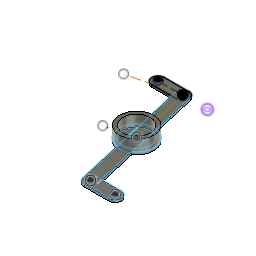
100x100 Naca 0012 airfoil w 3.8mm holes (Autodesk Fusion 360 design; units mm, degrees)
Autodesk Fusion 360 part; units mm, degrees
sketch "NACA_0012_AIRFOILS_1.0" plane through (0, 0, 0) normal (0, 0, 1) x (1, 0, 0)
  spline S0 degree 5 poles (100, 0.126) (99.9938, 0.1269) (99.9778, 0.1291) (99.9427, 0.134) (99.8738, 0.1437) (99.7628, 0.1592) (99.6406, 0.1763) (99.5101, 0.1946) (99.3691, 0.2142) (99.2177, 0.2353) (99.0577, 0.2575) (98.8912, 0.2806) (98.7187, 0.3044) (98.5403, 0.3289) (98.356, 0.3543) (98.166, 0.3804) (97.9707, 0.4072) (97.7707, 0.4346) (97.5662, 0.4625) (97.3575, 0.4909) (97.1446, 0.5198) (96.9277, 0.5491) (96.7068, 0.5789) (96.4822, 0.6091) (96.254, 0.6397) (96.0224, 0.6708) (95.7875, 0.7021) (95.5493, 0.7338) (95.3081, 0.7658) (95.0637, 0.7982) (94.8164, 0.8308) (94.5663, 0.8637) (94.3133, 0.8969) (94.0576, 0.9304) (93.7993, 0.9641) (93.5384, 0.998) (93.275, 1.0321) (93.0091, 1.0665) (92.7408, 1.101) (92.4702, 1.1357) (92.1973, 1.1706) (91.9221, 1.2057) (91.6448, 1.2409) (91.3653, 1.2763) (91.0838, 1.3119) (90.8001, 1.3476) (90.5145, 1.3835) (90.2269, 1.4194) (89.9374, 1.4555) (89.646, 1.4917) (89.3527, 1.528) (89.0576, 1.5644) (88.7607, 1.6009) (88.4621, 1.6375) (88.1617, 1.6742) (87.8597, 1.7109) (87.556, 1.7477) (87.2507, 1.7846) (86.9439, 1.8216) (86.6354, 1.8586) (86.3255, 1.8956) (86.014, 1.9327) (85.701, 1.9699) (85.3866, 2.0071) (85.0707, 2.0443) (84.7534, 2.0816) (84.4348, 2.1188) (84.1147, 2.1561) (83.7934, 2.1934) (83.4707, 2.2307) (83.1468, 2.268) (82.8216, 2.3053) (82.4952, 2.3426) (82.1675, 2.3799) (81.8386, 2.4172) (81.5086, 2.4545) (81.1774, 2.4918) (80.845, 2.5291) (80.5115, 2.5664) (80.1769, 2.6036) (79.8413, 2.6408) (79.5046, 2.6779) (79.1668, 2.715) (78.828, 2.7521) (78.4882, 2.7891) (78.1474, 2.8261) (77.8056, 2.863) (77.4628, 2.8999) (77.1192, 2.9368) (76.7745, 2.9735) (76.429, 3.0103) (76.0826, 3.0469) (75.7353, 3.0835) (75.3872, 3.1199) (75.0382, 3.1564) (74.6884, 3.1927) (74.3377, 3.229) (73.9863, 3.2652) (73.634, 3.3013) (73.281, 3.3373) (72.9273, 3.3732) (72.5728, 3.4091) (72.2175, 3.4448) (71.8616, 3.4805) (71.5049, 3.516) (71.1476, 3.5514) (70.7896, 3.5867) (70.4309, 3.6219) (70.0716, 3.657) (69.7117, 3.6919) (69.3511, 3.7268) (68.99, 3.7615) (68.6282, 3.7961) (68.2659, 3.8306) (67.903, 3.8649) (67.5395, 3.8991) (67.1755, 3.9331) (66.811, 3.967) (66.4459, 4.0007) (66.0804, 4.0343) (65.7143, 4.0678) (65.3478, 4.1011) (64.9808, 4.1342) (64.6134, 4.1672) (64.2455, 4.2001) (63.8771, 4.2327) (63.5084, 4.2652) (63.1392, 4.2975) (62.7697, 4.3296) (62.3997, 4.3616) (62.0294, 4.3933) (61.6587, 4.4249) (61.2877, 4.4563) (60.9163, 4.4874) (60.5447, 4.5184) (60.1726, 4.5492) (59.8003, 4.5798) (59.4277, 4.6101) (59.0549, 4.6403) (58.6817, 4.6702) (58.3083, 4.7) (57.9346, 4.7295) (57.5607, 4.7588) (57.1865, 4.7878) (56.8122, 4.8166) (56.4376, 4.8452) (56.0628, 4.8736) (55.6879, 4.9016) (55.3128, 4.9295) (54.9375, 4.9571) (54.5621, 4.9844) (54.1865, 5.0115) (53.8108, 5.0383) (53.435, 5.0648) (53.0591, 5.0911) (52.6831, 5.1171) (52.307, 5.1428) (51.9308, 5.1682) (51.5545, 5.1934) (51.1782, 5.2182) (50.8019, 5.2428) (50.4255, 5.2671) (50.0491, 5.291) (49.6727, 5.3147) (49.2963, 5.338) (48.9199, 5.361) (48.5435, 5.3837) (48.1672, 5.4061) (47.7909, 5.4281) (47.4146, 5.4498) (47.0384, 5.4711) (46.6623, 5.4922) (46.2863, 5.5128) (45.9104, 5.5331) (45.5345, 5.5531) (45.1588, 5.5727) (44.7833, 5.5919) (44.4078, 5.6107) (44.0326, 5.6292) (43.6574, 5.6473) (43.2825, 5.665) (42.9077, 5.6823) (42.5332, 5.6992) (42.1588, 5.7157) (41.7847, 5.7319) (41.4108, 5.7475) (41.0371, 5.7628) (40.6637, 5.7777) (40.2905, 5.7921) (39.9177, 5.8061) (39.5451, 5.8197) (39.1728, 5.8328) (38.8008, 5.8455) (38.4291, 5.8578) (38.0578, 5.8695) (37.6868, 5.8809) (37.3162, 5.8917) (36.9459, 5.9021) (36.576, 5.912) (36.2065, 5.9214) (35.8375, 5.9303) (35.4688, 5.9388) (35.1006, 5.9467) (34.7328, 5.9541) (34.3654, 5.961) (33.9986, 5.9674) (33.6322, 5.9733) (33.2662, 5.9786) (32.9008, 5.9834) (32.536, 5.9877) (32.1716, 5.9914) (31.8078, 5.9945) (31.4445, 5.9971) (31.0818, 5.9992) (30.7197, 6.0007) (30.3582, 6.0015) (29.9973, 6.0019) (29.637, 6.0016) (29.2774, 6.0007) (28.9184, 5.9992) (28.5601, 5.9972) (28.2024, 5.9945) (27.8455, 5.9912) (27.4892, 5.9873) (27.1337, 5.9828) (26.779, 5.9776) (26.4249, 5.9718) (26.0717, 5.9653) (25.7192, 5.9582) (25.3676, 5.9504) (25.0167, 5.9419) (24.6667, 5.9327) (24.3176, 5.9229) (23.9693, 5.9123) (23.6219, 5.9011) (23.2754, 5.8892) (22.9298, 5.8766) (22.5851, 5.8632) (22.2414, 5.8492) (21.8987, 5.8344) (21.5569, 5.8188) (21.2162, 5.8026) (20.8764, 5.7855) (20.5378, 5.7677) (20.2001, 5.7492) (19.8636, 5.7298) (19.5282, 5.7097) (19.1939, 5.6888) (18.8607, 5.6671) (18.5287, 5.6446) (18.1979, 5.6213) (17.8683, 5.5971) (17.5399, 5.5721) (17.2127, 5.5463) (16.8869, 5.5197) (16.5623, 5.4922) (16.2391, 5.4638) (15.9172, 5.4345) (15.5967, 5.4043) (15.2776, 5.3733) (14.9599, 5.3414) (14.6437, 5.3085) (14.3289, 5.2747) (14.0157, 5.24) (13.704, 5.2043) (13.3938, 5.1677) (13.0852, 5.1302) (12.7783, 5.0916) (12.473, 5.0521) (12.1694, 5.0116) (11.8675, 4.9701) (11.5673, 4.9276) (11.269, 4.884) (10.9725, 4.8394) (10.6779, 4.7937) (10.3851, 4.7469) (10.0943, 4.699) (9.8055, 4.65) (9.5187, 4.5999) (9.234, 4.5486) (8.9514, 4.4962) (8.6709, 4.4426) (8.3927, 4.3878) (8.1167, 4.3318) (7.843, 4.2746) (7.5717, 4.2161) (7.3029, 4.1564) (7.0365, 4.0953) (6.7727, 4.0329) (6.5114, 3.9691) (6.2529, 3.9039) (5.9971, 3.8373) (5.7442, 3.7693) (5.4941, 3.6998) (5.247, 3.6288) (5.0031, 3.5562) (4.7622, 3.4821) (4.5247, 3.4063) (4.2905, 3.3288) (4.0599, 3.2495) (3.8328, 3.1685) (3.6094, 3.0857) (3.39, 3.0009) (3.1745, 2.9142) (2.9632, 2.8254) (2.7563, 2.7345) (2.5539, 2.6415) (2.3562, 2.5461) (2.1635, 2.4483) (1.976, 2.3481) (1.794, 2.2452) (1.6177, 2.1397) (1.4475, 2.0313) (1.2838, 1.9199) (1.1269, 1.8055) (0.9774, 1.6878) (0.8357, 1.5667) (0.7024, 1.442) (0.5781, 1.3137) (0.4636, 1.1815) (0.3595, 1.0456) (0.2668, 0.9058) (0.1864, 0.7624) (0.1191, 0.6153) (0.0658, 0.4649) (0.0272, 0.3117) (0.0039, 0.1564) (-0.0039, 0) (0.0039, -0.1564) (0.0272, -0.3117) (0.0658, -0.4649) (0.1191, -0.6153) (0.1864, -0.7624) (0.2668, -0.9058) (0.3595, -1.0456) (0.4636, -1.1815) (0.5781, -1.3137) (0.7024, -1.442) (0.8357, -1.5667) (0.9774, -1.6878) (1.1269, -1.8055) (1.2838, -1.9199) (1.4475, -2.0313) (1.6177, -2.1397) (1.794, -2.2452) (1.976, -2.3481) (2.1635, -2.4483) (2.3562, -2.5461) (2.5539, -2.6415) (2.7563, -2.7345) (2.9632, -2.8254) (3.1745, -2.9142) (3.39, -3.0009) (3.6094, -3.0857) (3.8328, -3.1685) (4.0599, -3.2495) (4.2905, -3.3288) (4.5247, -3.4063) (4.7622, -3.4821) (5.0031, -3.5562) (5.247, -3.6288) (5.4941, -3.6998) (5.7442, -3.7693) (5.9971, -3.8373) (6.2529, -3.9039) (6.5114, -3.9691) (6.7727, -4.0329) (7.0365, -4.0953) (7.3029, -4.1564) (7.5717, -4.2161) (7.843, -4.2746) (8.1167, -4.3318) (8.3927, -4.3878) (8.6709, -4.4426) (8.9514, -4.4962) (9.234, -4.5486) (9.5187, -4.5999) (9.8055, -4.65) (10.0943, -4.699) (10.3851, -4.7469) (10.6779, -4.7937) (10.9725, -4.8394) (11.269, -4.884) (11.5673, -4.9276) (11.8675, -4.9701) (12.1694, -5.0116) (12.473, -5.0521) (12.7783, -5.0916) (13.0852, -5.1302) (13.3938, -5.1677) (13.704, -5.2043) (14.0157, -5.24) (14.3289, -5.2747) (14.6437, -5.3085) (14.9599, -5.3414) (15.2776, -5.3733) (15.5967, -5.4043) (15.9172, -5.4345) (16.2391, -5.4638) (16.5623, -5.4922) (16.8869, -5.5197) (17.2127, -5.5463) (17.5399, -5.5721) (17.8683, -5.5971) (18.1979, -5.6213) (18.5287, -5.6446) (18.8607, -5.6671) (19.1939, -5.6888) (19.5282, -5.7097) (19.8636, -5.7298) (20.2001, -5.7492) (20.5378, -5.7677) (20.8764, -5.7855) (21.2162, -5.8026) (21.5569, -5.8188) (21.8987, -5.8344) (22.2414, -5.8492) (22.5851, -5.8632) (22.9298, -5.8766) (23.2754, -5.8892) (23.6219, -5.9011) (23.9693, -5.9123) (24.3176, -5.9229) (24.6667, -5.9327) (25.0167, -5.9419) (25.3676, -5.9504) (25.7192, -5.9582) (26.0717, -5.9653) (26.4249, -5.9718) (26.779, -5.9776) (27.1337, -5.9828) (27.4892, -5.9873) (27.8455, -5.9912) (28.2024, -5.9945) (28.5601, -5.9972) (28.9184, -5.9992) (29.2774, -6.0007) (29.637, -6.0016) (29.9973, -6.0019) (30.3582, -6.0015) (30.7197, -6.0007) (31.0818, -5.9992) (31.4445, -5.9971) (31.8078, -5.9945) (32.1716, -5.9914) (32.536, -5.9877) (32.9008, -5.9834) (33.2662, -5.9786) (33.6322, -5.9733) (33.9986, -5.9674) (34.3654, -5.961) (34.7328, -5.9541) (35.1006, -5.9467) (35.4688, -5.9388) (35.8375, -5.9303) (36.2065, -5.9214) (36.576, -5.912) (36.9459, -5.9021) (37.3162, -5.8917) (37.6868, -5.8809) (38.0578, -5.8695) (38.4291, -5.8578) (38.8008, -5.8455) (39.1728, -5.8328) (39.5451, -5.8197) (39.9177, -5.8061) (40.2905, -5.7921) (40.6637, -5.7777) (41.0371, -5.7628) (41.4108, -5.7475) (41.7847, -5.7319) (42.1588, -5.7157) (42.5332, -5.6992) (42.9077, -5.6823) (43.2825, -5.665) (43.6574, -5.6473) (44.0326, -5.6292) (44.4078, -5.6107) (44.7833, -5.5919) (45.1588, -5.5727) (45.5345, -5.5531) (45.9104, -5.5331) (46.2863, -5.5128) (46.6623, -5.4922) (47.0384, -5.4711) (47.4146, -5.4498) (47.7909, -5.4281) (48.1672, -5.4061) (48.5435, -5.3837) (48.9199, -5.361) (49.2963, -5.338) (49.6727, -5.3147) (50.0491, -5.291) (50.4255, -5.2671) (50.8019, -5.2428) (51.1782, -5.2182) (51.5545, -5.1934) (51.9308, -5.1682) (52.307, -5.1428) (52.6831, -5.1171) (53.0591, -5.0911) (53.435, -5.0648) (53.8108, -5.0383) (54.1865, -5.0115) (54.5621, -4.9844) (54.9375, -4.9571) (55.3128, -4.9295) (55.6879, -4.9016) (56.0628, -4.8736) (56.4376, -4.8452) (56.8122, -4.8166) (57.1865, -4.7878) (57.5607, -4.7588) (57.9346, -4.7295) (58.3083, -4.7) (58.6817, -4.6702) (59.0549, -4.6403) (59.4277, -4.6101) (59.8003, -4.5798) (60.1726, -4.5492) (60.5447, -4.5184) (60.9163, -4.4874) (61.2877, -4.4563) (61.6587, -4.4249) (62.0294, -4.3933) (62.3997, -4.3616) (62.7697, -4.3296) (63.1392, -4.2975) (63.5084, -4.2652) (63.8771, -4.2327) (64.2455, -4.2001) (64.6134, -4.1672) (64.9808, -4.1342) (65.3478, -4.1011) (65.7143, -4.0678) (66.0804, -4.0343) (66.4459, -4.0007) (66.811, -3.967) (67.1755, -3.9331) (67.5395, -3.8991) (67.903, -3.8649) (68.2659, -3.8306) (68.6282, -3.7961) (68.99, -3.7615) (69.3511, -3.7268) (69.7117, -3.6919) (70.0716, -3.657) (70.4309, -3.6219) (70.7896, -3.5867) (71.1476, -3.5514) (71.5049, -3.516) (71.8616, -3.4805) (72.2175, -3.4448) (72.5728, -3.4091) (72.9273, -3.3732) (73.281, -3.3373) (73.634, -3.3013) (73.9863, -3.2652) (74.3377, -3.229) (74.6884, -3.1927) (75.0382, -3.1564) (75.3872, -3.1199) (75.7353, -3.0835) (76.0826, -3.0469) (76.429, -3.0103) (76.7745, -2.9735) (77.1192, -2.9368) (77.4628, -2.8999) (77.8056, -2.863) (78.1474, -2.8261) (78.4882, -2.7891) (78.828, -2.7521) (79.1668, -2.715) (79.5046, -2.6779) (79.8413, -2.6408) (80.1769, -2.6036) (80.5115, -2.5664) (80.845, -2.5291) (81.1774, -2.4918) (81.5086, -2.4545) (81.8386, -2.4172) (82.1675, -2.3799) (82.4952, -2.3426) (82.8216, -2.3053) (83.1468, -2.268) (83.4707, -2.2307) (83.7934, -2.1934) (84.1147, -2.1561) (84.4348, -2.1188) (84.7534, -2.0816) (85.0707, -2.0443) (85.3866, -2.0071) (85.701, -1.9699) (86.014, -1.9327) (86.3255, -1.8956) (86.6354, -1.8586) (86.9439, -1.8216) (87.2507, -1.7846) (87.556, -1.7477) (87.8597, -1.7109) (88.1617, -1.6742) (88.4621, -1.6375) (88.7607, -1.6009) (89.0576, -1.5644) (89.3527, -1.528) (89.646, -1.4917) (89.9374, -1.4555) (90.2269, -1.4194) (90.5145, -1.3835) (90.8001, -1.3476) (91.0838, -1.3119) (91.3653, -1.2763) (91.6448, -1.2409) (91.9221, -1.2057) (92.1973, -1.1706) (92.4702, -1.1357) (92.7408, -1.101) (93.0091, -1.0665) (93.275, -1.0321) (93.5384, -0.998) (93.7993, -0.9641) (94.0576, -0.9304) (94.3133, -0.8969) (94.5663, -0.8637) (94.8164, -0.8308) (95.0637, -0.7982) (95.3081, -0.7658) (95.5493, -0.7338) (95.7875, -0.7021) (96.0224, -0.6708) (96.254, -0.6397) (96.4822, -0.6091) (96.7068, -0.5789) (96.9277, -0.5491) (97.1446, -0.5198) (97.3575, -0.4909) (97.5662, -0.4625) (97.7707, -0.4346) (97.9707, -0.4072) (98.166, -0.3804) (98.356, -0.3543) (98.5403, -0.3289) (98.7187, -0.3044) (98.8912, -0.2806) (99.0577, -0.2575) (99.2177, -0.2353) (99.3691, -0.2142) (99.5101, -0.1946) (99.6406, -0.1763) (99.7628, -0.1592) (99.8738, -0.1437) (99.9427, -0.134) (99.9778, -0.1291) (99.9938, -0.1269) (100, -0.126) knots 0 0 0 0 0 0 0.00153846 0.00307692 0.00461538 0.00615385 0.00769231 0.00923077 0.01076923 0.01230769 0.01384615 0.01538462 0.01692308 0.01846154 0.02 0.02153846 0.02307692 0.02461538 0.02615385 0.02769231 0.02923077 0.03076923 0.03230769 0.03384615 0.03538462 0.03692308 0.03846154 0.04 0.04153846 0.04307692 0.04461538 0.04615385 0.04769231 0.04923077 0.05076923 0.05230769 0.05384615 0.05538462 0.05692308 0.05846154 0.06 0.06153846 0.06307692 0.06461538 0.06615385 0.06769231 0.06923077 0.07076923 0.07230769 0.07384615 0.07538462 0.07692308 0.07846154 0.08 0.08153846 0.08307692 0.08461538 0.08615385 0.08769231 0.08923077 0.09076923 0.09230769 0.09384615 0.09538462 0.09692308 0.09846154 0.1 0.10153846 0.10307692 0.10461538 0.10615385 0.10769231 0.10923077 0.11076923 0.11230769 0.11384615 0.11538462 0.11692308 0.11846154 0.12 0.12153846 0.12307692 0.12461538 0.12615385 0.12769231 0.12923077 0.13076923 0.13230769 0.13384615 0.13538462 0.13692308 0.13846154 0.14 0.14153846 0.14307692 0.14461538 0.14615385 0.14769231 0.14923077 0.15076923 0.15230769 0.15384615 0.15538462 0.15692308 0.15846154 0.16 0.16153846 0.16307692 0.16461538 0.16615385 0.16769231 0.16923077 0.17076923 0.17230769 0.17384615 0.17538462 0.17692308 0.17846154 0.18 0.18153846 0.18307692 0.18461538 0.18615385 0.18769231 0.18923077 0.19076923 0.19230769 0.19384615 0.19538462 0.19692308 0.19846154 0.2 0.20153846 0.20307692 0.20461538 0.20615385 0.20769231 0.20923077 0.21076923 0.21230769 0.21384615 0.21538462 0.21692308 0.21846154 0.22 0.22153846 0.22307692 0.22461538 0.22615385 0.22769231 0.22923077 0.23076923 0.23230769 0.23384615 0.23538462 0.23692308 0.23846154 0.24 0.24153846 0.24307692 0.24461538 0.24615385 0.24769231 0.24923077 0.25076923 0.25230769 0.25384615 0.25538462 0.25692308 0.25846154 0.26 0.26153846 0.26307692 0.26461538 0.26615385 0.26769231 0.26923077 0.27076923 0.27230769 0.27384615 0.27538462 0.27692308 0.27846154 0.28 0.28153846 0.28307692 0.28461538 0.28615385 0.28769231 0.28923077 0.29076923 0.29230769 0.29384615 0.29538462 0.29692308 0.29846154 0.3 0.30153846 0.30307692 0.30461538 0.30615385 0.30769231 0.30923077 0.31076923 0.31230769 0.31384615 0.31538462 0.31692308 0.31846154 0.32 0.32153846 0.32307692 0.32461538 0.32615385 0.32769231 0.32923077 0.33076923 0.33230769 0.33384615 0.33538462 0.33692308 0.33846154 0.34 0.34153846 0.34307692 0.34461538 0.34615385 0.34769231 0.34923077 0.35076923 0.35230769 0.35384615 0.35538462 0.35692308 0.35846154 0.36 0.36153846 0.36307692 0.36461538 0.36615385 0.36769231 0.36923077 0.37076923 0.37230769 0.37384615 0.37538462 0.37692308 0.37846154 0.38 0.38153846 0.38307692 0.38461538 0.38615385 0.38769231 0.38923077 0.39076923 0.39230769 0.39384615 0.39538462 0.39692308 0.39846154 0.4 0.40153846 0.40307692 0.40461538 0.40615385 0.40769231 0.40923077 0.41076923 0.41230769 0.41384615 0.41538462 0.41692308 0.41846154 0.42 0.42153846 0.42307692 0.42461538 0.42615385 0.42769231 0.42923077 0.43076923 0.43230769 0.43384615 0.43538462 0.43692308 0.43846154 0.44 0.44153846 0.44307692 0.44461538 0.44615385 0.44769231 0.44923077 0.45076923 0.45230769 0.45384615 0.45538462 0.45692308 0.45846154 0.46 0.46153846 0.46307692 0.46461538 0.46615385 0.46769231 0.46923077 0.47076923 0.47230769 0.47384615 0.47538462 0.47692308 0.47846154 0.48 0.48153846 0.48307692 0.48461538 0.48615385 0.48769231 0.48923077 0.49076923 0.49230769 0.49384615 0.49538462 0.49692308 0.49846154 0.5 0.50153846 0.50307692 0.50461538 0.50615385 0.50769231 0.50923077 0.51076923 0.51230769 0.51384615 0.51538462 0.51692308 0.51846154 0.52 0.52153846 0.52307692 0.52461538 0.52615385 0.52769231 0.52923077 0.53076923 0.53230769 0.53384615 0.53538462 0.53692308 0.53846154 0.54 0.54153846 0.54307692 0.54461538 0.54615385 0.54769231 0.54923077 0.55076923 0.55230769 0.55384615 0.55538462 0.55692308 0.55846154 0.56 0.56153846 0.56307692 0.56461538 0.56615385 0.56769231 0.56923077 0.57076923 0.57230769 0.57384615 0.57538462 0.57692308 0.57846154 0.58 0.58153846 0.58307692 0.58461538 0.58615385 0.58769231 0.58923077 0.59076923 0.59230769 0.59384615 0.59538462 0.59692308 0.59846154 0.6 0.60153846 0.60307692 0.60461538 0.60615385 0.60769231 0.60923077 0.61076923 0.61230769 0.61384615 0.61538462 0.61692308 0.61846154 0.62 0.62153846 0.62307692 0.62461538 0.62615385 0.62769231 0.62923077 0.63076923 0.63230769 0.63384615 0.63538462 0.63692308 0.63846154 0.64 0.64153846 0.64307692 0.64461538 0.64615385 0.64769231 0.64923077 0.65076923 0.65230769 0.65384615 0.65538462 0.65692308 0.65846154 0.66 0.66153846 0.66307692 0.66461538 0.66615385 0.66769231 0.66923077 0.67076923 0.67230769 0.67384615 0.67538462 0.67692308 0.67846154 0.68 0.68153846 0.68307692 0.68461538 0.68615385 0.68769231 0.68923077 0.69076923 0.69230769 0.69384615 0.69538462 0.69692308 0.69846154 0.7 0.70153846 0.70307692 0.70461538 0.70615385 0.70769231 0.70923077 0.71076923 0.71230769 0.71384615 0.71538462 0.71692308 0.71846154 0.72 0.72153846 0.72307692 0.72461538 0.72615385 0.72769231 0.72923077 0.73076923 0.73230769 0.73384615 0.73538462 0.73692308 0.73846154 0.74 0.74153846 0.74307692 0.74461538 0.74615385 0.74769231 0.74923077 0.75076923 0.75230769 0.75384615 0.75538462 0.75692308 0.75846154 0.76 0.76153846 0.76307692 0.76461538 0.76615385 0.76769231 0.76923077 0.77076923 0.77230769 0.77384615 0.77538462 0.77692308 0.77846154 0.78 0.78153846 0.78307692 0.78461538 0.78615385 0.78769231 0.78923077 0.79076923 0.79230769 0.79384615 0.79538462 0.79692308 0.79846154 0.8 0.80153846 0.80307692 0.80461538 0.80615385 0.80769231 0.80923077 0.81076923 0.81230769 0.81384615 0.81538462 0.81692308 0.81846154 0.82 0.82153846 0.82307692 0.82461538 0.82615385 0.82769231 0.82923077 0.83076923 0.83230769 0.83384615 0.83538462 0.83692308 0.83846154 0.84 0.84153846 0.84307692 0.84461538 0.84615385 0.84769231 0.84923077 0.85076923 0.85230769 0.85384615 0.85538462 0.85692308 0.85846154 0.86 0.86153846 0.86307692 0.86461538 0.86615385 0.86769231 0.86923077 0.87076923 0.87230769 0.87384615 0.87538462 0.87692308 0.87846154 0.88 0.88153846 0.88307692 0.88461538 0.88615385 0.88769231 0.88923077 0.89076923 0.89230769 0.89384615 0.89538462 0.89692308 0.89846154 0.9 0.90153846 0.90307692 0.90461538 0.90615385 0.90769231 0.90923077 0.91076923 0.91230769 0.91384615 0.91538462 0.91692308 0.91846154 0.92 0.92153846 0.92307692 0.92461538 0.92615385 0.92769231 0.92923077 0.93076923 0.93230769 0.93384615 0.93538462 0.93692308 0.93846154 0.94 0.94153846 0.94307692 0.94461538 0.94615385 0.94769231 0.94923077 0.95076923 0.95230769 0.95384615 0.95538462 0.95692308 0.95846154 0.96 0.96153846 0.96307692 0.96461538 0.96615385 0.96769231 0.96923077 0.97076923 0.97230769 0.97384615 0.97538462 0.97692308 0.97846154 0.98 0.98153846 0.98307692 0.98461538 0.98615385 0.98769231 0.98923077 0.99076923 0.99230769 0.99384615 0.99538462 0.99692308 0.99846154 1 1 1 1 1 1
  line L0 (100, -0.126) -> (100, 0.126)
  line L1 (0, 0) -> (100, 0) construction
  circle A0 centre (30, 0) radius 1.9
  point P0 (99.9416, 0.1342)
  point P1 (99.7666, 0.1587)
  point P2 (99.4753, 0.1994)
  point P3 (99.0685, 0.256)
  point P4 (98.5471, 0.328)
  point P5 (97.9123, 0.4152)
  point P6 (97.1656, 0.5169)
  point P7 (96.3087, 0.6324)
  point P8 (95.3437, 0.7611)
  point P9 (94.2728, 0.9022)
  point P10 (93.0985, 1.0549)
  point P11 (91.8235, 1.2182)
  point P12 (90.4509, 1.3914)
  point P13 (88.9837, 1.5735)
  point P14 (87.4255, 1.7635)
  point P15 (85.78, 1.9605)
  point P16 (84.0508, 2.1635)
  point P17 (82.2421, 2.3714)
  point P18 (80.3581, 2.5834)
  point P19 (78.4032, 2.7983)
  point P20 (76.382, 3.0152)
  point P21 (74.2992, 3.2329)
  point P22 (72.1596, 3.4506)
  point P23 (69.9682, 3.667)
  point P24 (67.7303, 3.8811)
  point P25 (65.4509, 4.0917)
  point P26 (63.1354, 4.2978)
  point P27 (60.7892, 4.498)
  point P28 (58.4179, 4.6912)
  point P29 (56.0268, 4.8762)
  point P30 (53.6217, 5.0516)
  point P31 (51.2082, 5.2162)
  point P32 (48.7918, 5.3687)
  point P33 (46.3783, 5.5077)
  point P34 (43.9732, 5.632)
  point P35 (41.5822, 5.7403)
  point P36 (39.2108, 5.8314)
  point P37 (36.8646, 5.9042)
  point P38 (34.5492, 5.9575)
  point P39 (32.2698, 5.9903)
  point P40 (30.0318, 6.0017)
  point P41 (27.8404, 5.991)
  point P42 (25.7008, 5.9576)
  point P43 (23.618, 5.9008)
  point P44 (21.5968, 5.8205)
  point P45 (19.6419, 5.7164)
  point P46 (17.7579, 5.5886)
  point P47 (15.9492, 5.4372)
  point P48 (14.2201, 5.2625)
  point P49 (12.5745, 5.0651)
  point P50 (11.0163, 4.8457)
  point P51 (9.5492, 4.6049)
  point P52 (8.1765, 4.3437)
  point P53 (6.9015, 4.0631)
  point P54 (5.7272, 3.7641)
  point P55 (4.6563, 3.4479)
  point P56 (3.6913, 3.1156)
  point P57 (2.8344, 2.7683)
  point P58 (2.0877, 2.4071)
  point P59 (1.4529, 2.033)
  point P60 (0.9315, 1.6471)
  point P61 (0.5247, 1.2501)
  point P62 (0.2334, 0.8429)
  point P63 (0.0584, 0.426)
  point P64 (0.0584, -0.426)
  point P65 (0.2334, -0.8429)
  point P66 (0.5247, -1.2501)
  point P67 (0.9315, -1.6471)
  point P68 (1.4529, -2.033)
  point P69 (2.0877, -2.4071)
  point P70 (2.8344, -2.7683)
  point P71 (3.6913, -3.1156)
  point P72 (4.6563, -3.4479)
  point P73 (5.7272, -3.7641)
  point P74 (6.9015, -4.0631)
  point P75 (8.1765, -4.3437)
  point P76 (9.5492, -4.6049)
  point P77 (11.0163, -4.8457)
  point P78 (12.5745, -5.0651)
  point P79 (14.2201, -5.2625)
  point P80 (15.9492, -5.4372)
  point P81 (17.7579, -5.5886)
  point P82 (19.6419, -5.7164)
  point P83 (21.5968, -5.8205)
  point P84 (23.618, -5.9008)
  point P85 (25.7008, -5.9576)
  point P86 (27.8404, -5.991)
  point P87 (30.0318, -6.0017)
  point P88 (32.2698, -5.9903)
  point P89 (34.5492, -5.9575)
  point P90 (36.8646, -5.9042)
  point P91 (39.2108, -5.8314)
  point P92 (41.5822, -5.7403)
  point P93 (43.9732, -5.632)
  point P94 (46.3783, -5.5077)
  point P95 (48.7918, -5.3687)
  point P96 (51.2082, -5.2162)
  point P97 (53.6217, -5.0516)
  point P98 (56.0268, -4.8762)
  point P99 (58.4179, -4.6912)
  point P100 (60.7892, -4.498)
  point P101 (63.1354, -4.2978)
  point P102 (65.4509, -4.0917)
  point P103 (67.7303, -3.8811)
  point P104 (69.9682, -3.667)
  point P105 (72.1596, -3.4506)
  point P106 (74.2992, -3.2329)
  point P107 (76.382, -3.0152)
  point P108 (78.4032, -2.7983)
  point P109 (80.3581, -2.5834)
  point P110 (82.2421, -2.3714)
  point P111 (84.0508, -2.1635)
  point P112 (85.78, -1.9605)
  point P113 (87.4255, -1.7635)
  point P114 (88.9837, -1.5735)
  point P115 (90.4509, -1.3914)
  point P116 (91.8235, -1.2182)
  point P117 (93.0985, -1.0549)
  point P118 (94.2728, -0.9022)
  point P119 (95.3437, -0.7611)
  point P120 (96.3087, -0.6324)
  point P121 (97.1656, -0.5169)
  point P122 (97.9123, -0.4152)
  point P123 (98.5471, -0.328)
  point P124 (99.0685, -0.256)
  point P125 (99.4753, -0.1994)
  point P126 (99.7666, -0.1587)
  point P127 (99.9416, -0.1342)
  dimension "d3" = 100
  dimension "d4" = 30
  dimension "d5" = 3.8
  constraint vertical L0
  constraint coincident L1.start origin
  constraint midpoint L0 L1.end
  constraint coincident L1 A0.centre
  measures "d3" distance of L1.start L1.end
  measures "d4" distance of L1.start A0.centre
  measures "d5" diameter of A0
extrude "Extrude1" add sketch "NACA_0012_AIRFOILS_1.0" along normal blind 100 contours S0 L0 | A0 makes body 1
sketch "Sketch2" plane through (0, 0, 0) normal (0, 0, 1) x (1, 0, 0)
  line L0 (0, 0) -> (100, 0) construction
  circle A0 centre (10, 0) radius 1.9
  circle A1 centre (50, 0) radius 1.9
  circle A2 centre (30, 0) radius 1.9
  dimension "d10" = 3.8
  dimension "d16" = 20
  dimension "d17" = 20
  constraint coincident L0 A0.centre
  constraint coincident L0 A1.centre
  constraint equal A0 A1
  measures "d10" diameter of A1
  measures "d16" distance of A0.centre A2.centre
  measures "d17" distance of A1.centre A2.centre
extrude "Extrude3" cut sketch "Sketch2" sketch "NACA_0012_AIRFOILS_1.0" along normal blind 10 contours A0 | A1 of sketch 2 contours A0 bodies 1
extrude "Extrude4" cut sketch "Sketch2" sketch "NACA_0012_AIRFOILS_1.0" against normal blind 10 contours A0 | A1 of sketch 2 contours A0 start surface through (0, 0, 100) normal (0, 0, 1) bodies 1
copy_body "Body->Comp1" bodies 1 removing the originals makes body 2 in component "100x100 Naca 0012 airfoil w 3.8mm holes"
sketch "Connecting Bar 13 degree 100mm" plane through (0, 0, 0) normal (0, 0, 1) x (1, 0, 0) in component "Connecting Bar"
  circle A0 centre (30, 0) radius 1.9
  circle A1 centre (50, 0) radius 1.9
  circle A2 centre (10, 0) radius 1.9
  line L0 (30, 0) -> (41.2476, -48.7185) construction
  line L1 (30, 0) -> (-9.0105, -9.0063) construction
  line L2 (10, -5) -> (26.0228, -5)
  line L3 (30, 5) -> (10, 5)
  arc A3 (10, 5) -> (10, -5) centre (10, 0) ccw
  line L4 (10, 0) -> (30, 0) construction
  line L5 (52.4951, -97.437) -> (30, 0) construction
  line L6 (41.2476, -48.7185) -> (18.862, -53.8866) construction
  line L7 (52.4951, -102.437) -> (72.4951, -102.437)
  arc A4 (72.4951, -102.437) -> (72.4951, -92.437) centre (72.4951, -97.437) ccw
  line L8 (72.4951, -92.437) -> (56.4723, -92.437)
  line L9 (52.4951, -97.437) -> (72.4951, -97.437) construction
  circle A5 centre (52.4951, -97.437) radius 1.9
  circle A6 centre (72.4951, -97.437) radius 1.9
  arc A7 (47.6233, -98.5618) -> (52.4951, -102.437) centre (52.4951, -97.437) ccw construction
  arc A8 (57.4951, -97.437) -> (57.367, -96.3123) centre (52.4951, -97.437) ccw construction
  arc A9 (52.4951, -102.437) -> (57.4951, -97.437) centre (52.4951, -97.437) ccw construction
  line L10 (57.367, -96.3123) -> (57.3106, -96.068)
  line L11 (57.3106, -96.068) -> (56.4723, -92.437)
  arc A10 (30, -5) -> (31.1248, -4.8719) centre (30, 0) ccw construction
  arc A11 (34.922, 0.8798) -> (30, 5) centre (30, 0) ccw construction
  arc A12 (31.1248, -4.8719) -> (34.922, 0.8798) centre (30, 0) ccw construction
  line L12 (26.0228, -5) -> (30, -5) construction
  arc A13 (34.8719, 1.1248) -> (30, 5) centre (30, 0) ccw
  arc A14 (25, 0) -> (25.1281, -1.1248) centre (30, 0) ccw
  arc A15 (30, 5) -> (25, 0) centre (30, 0) ccw construction
  line L13 (25.1281, -1.1248) -> (25.1845, -1.369)
  line L14 (25.1845, -1.369) -> (26.0228, -5) construction
  line L15 (56.4723, -92.437) -> (52.4951, -92.437) construction
  arc A16 (52.4951, -92.437) -> (51.3704, -92.5652) centre (52.4951, -97.437) ccw
  arc A17 (47.5731, -98.3168) -> (52.4951, -102.437) centre (52.4951, -97.437) ccw
  arc A18 (51.3704, -92.5652) -> (47.5731, -98.3168) centre (52.4951, -97.437) ccw construction
  circle A19 centre (41.2476, -48.7185) radius 11
  circle A20 centre (41.2476, -48.7185) radius 14
  arc A21 (40.3477, -44.821) -> (42.1474, -52.616) centre (41.2476, -48.7185) ccw
  arc A22 (42.1474, -52.616) -> (40.3477, -44.821) centre (41.2476, -48.7185) ccw
  line L16 (56.4723, -92.437) -> (48.3235, -57.1406)
  line L17 (43.9153, -38.0469) -> (34.8719, 1.1248)
  line L18 (48.3235, -57.1406) -> (43.9153, -38.0469)
  line L19 (26.0228, -5) -> (36.3757, -49.8433)
  line L20 (38.5798, -59.3901) -> (47.6233, -98.5618)
  line L21 (36.3757, -49.8433) -> (38.5798, -59.3901)
  point P0 (41.2476, -48.7185)
  dimension "d21" = 10
  dimension "d22" = 10
  dimension "d24" = 10
  dimension "d25" = 22
  dimension "d26" = 8
  dimension "d27" = 28
  dimension "d32" = 100
  constraint coincident A0.centre L0.start
  constraint perpendicular L0 L1
  constraint tangent L2 A10
  constraint tangent L3 A10
  constraint parallel L2 L3
  constraint tangent L3 A3
  constraint tangent L2 A3
  constraint horizontal L4
  constraint coincident A2.centre A3.centre
  constraint tangent L10 A13
  constraint tangent A13 L13
  constraint parallel L10 L13
  constraint tangent A7 L13
  constraint tangent A7 L10
  constraint parallel L0 L5
  constraint midpoint L5 P0
  constraint perpendicular L6 L13
  constraint tangent L7 A4
  constraint tangent A4 L8
  constraint parallel L7 L8
  constraint tangent L8 A16
  constraint tangent L7 A16
  constraint horizontal L9
  constraint coincident L5.start L9.start
  constraint equal L4 L9
  constraint concentric A5 A7
  constraint concentric A4 A6
  constraint equal A5 A6
  constraint equal A2 A5
  constraint coincident L9 A8.start
  constraint concentric A7 A8
  constraint concentric A7 A9
  constraint coincident L0 A10.end
  constraint concentric A10 A11
  constraint concentric A10 A12
  constraint coincident L2.end L13
  constraint tangent A10 L12
  constraint coincident L4 A14.start
  constraint concentric A13 A14
  constraint concentric A13 A15
  constraint tangent A4 L15
  constraint coincident L5 A16.end
  constraint concentric A16 A17
  constraint concentric A16 A18
  constraint coincident P0 L0.end
  constraint concentric A19 A20
  constraint coincident L5 A21.end
  constraint coincident L0 A21.start
  constraint concentric A21 A22
  constraint coincident A19 L16.end
  constraint coincident A19 L17.start
  constraint coincident L6 L19.end
  constraint coincident A19 L20.start
  measures "d21" diameter of A10
  measures "d22" diameter of A13
  measures "d24" diameter of A4
  measures "d25" diameter of A19
  measures "d26" diameter of A21
  measures "d27" diameter of A20
  measures "d32" distance of A0.centre L5.start
extrude "Extrude1'" add sketch "Connecting Bar 13 degree 100mm" along normal blind 9 separate body contours A19 A20 L19 L20 | A19 A20 L17 L19 | A19 A20 L16 L17 | A19 A20 L16 L20 makes body 3 in component "Connecting Bar"
extrude "Extrude2" add sketch "Connecting Bar 13 degree 100mm" against normal blind 2 contours L2 L3 A3 A13 A20 L17 L19 | A19 A20 L19 L20 | A19 A20 L17 L19 | A19 A20 L16 L17 | A19 A20 L16 L20 | L7 A4 L8 A17 A20 L16 L20 | A19 L19 L21 | A19 L18 L19 L21 | A19 L18 bodies 3 in component "Connecting Bar"
component "100x100 Naca 0012 airfoil w 3.8mm holes" placed x (1, 0, 0) y (0, 1, 0) z (0, 0, 1) at (0, 0, 0)
component "Connecting Bar" placed x (1, 0, 0) y (0, 1, 0) z (0, 0, 1) at (0, 0, 0)
equation "d4 = d3 * 0.3"
named bodies: "100x100 Naca 0012 airfoil w 3.8mm holes"
